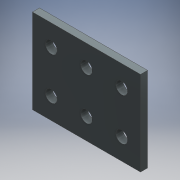
# Autodesk Inventor part: chassiconnector
Saved by Autodesk Inventor 2016 (Build 200138000, 138)
## iProperties
Created: 2017-01-05
Part Number: chassiconnector
Material: Generic
Document SubType Name: Modeling
Designer: hesaon
Density: 1 g/cm^3
Appearance: Default
Author: hesaon
Autodesk Inventor part; units mm, degrees
ref_plane "YZ Plane" through (0, 0, 0) normal (1, 0, 0) x (0, 1, 0)
ref_plane "XZ Plane" through (0, 0, 0) normal (0, 1, 0) x (-1, 0, 0)
ref_plane "XY Plane" through (0, 0, 0) normal (0, 0, 1) x (1, 0, 0)
sketch "Sketch1" plane through (0, 0, 0) normal (0, 1, 0) x (-1, 0, 0)
  line L0 (0, 0) -> (46, 0)
  line L1 (46, 0) -> (46, -36)
  line L2 (46, -36) -> (0, -36)
  line L3 (0, -36) -> (0, 0)
  circle A0 centre (38, -27) radius 2.5
  circle A1 centre (8, -27) radius 2.5
  circle A2 centre (23, -27) radius 2.5
  line L4 (46, -18) -> (0, -18)
  circle A3 centre (38, -9) radius 2.5
  circle A4 centre (8, -9) radius 2.5
  circle A5 centre (23, -9) radius 2.5
  dimension "d0" = 46
  dimension "d1" = 36
  dimension "d2" = 5
  dimension "d3" = 8
  dimension "d4" = 27
  dimension "d6" = 5
  dimension "d7" = 8
  dimension "d13" = 5
  dimension "d15" = 15
  constraints: 10 end point, 6 centre point, 3 symmetric about line, 2 horizontal alignment, 2 midpoint, 2 parallel, 1 horizontal, 1 perpendicular, 3 other
  measures "d0" distance of L1.end L2.end
  measures "d1" distance of L0.end L1.end
  measures "d2" diameter of A0
  measures "d3" distance from line of A0.centre L1
  measures "d4" distance from line of L0 A0.centre
  measures "d6" diameter of A1
  measures "d7" distance from line of L3 A1.centre
  measures "d13" diameter of A2
  measures "d15" distance of A2.centre A0.centre
extrude "Extrusion6" add sketch "Sketch1" along normal blind 3
body "Solid4"
